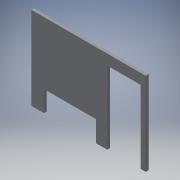
# Autodesk Inventor part: CANIMDWall
Saved by Autodesk Inventor 2017 (Build 210142000, 142)
## iProperties
Created: 2017-03-28
Part Number: CANIMDWall
Material: Generic
Document SubType Name: Modeling
Designer: hoeflinc
Density: 1 g/cm^3
Appearance: Default
Quantity: 1
Author: hoeflinc
Autodesk Inventor part; units mm, degrees
ref_plane "YZ Plane" through (0, 0, 0) normal (1, 0, 0) x (0, 1, 0)
ref_plane "XZ Plane" through (0, 0, 0) normal (0, 1, 0) x (-1, 0, 0)
ref_plane "XY Plane" through (0, 0, 0) normal (0, 0, 1) x (1, 0, 0)
sketch "Sketch1" plane through (0, 0, 0) normal (0, 0, 1) x (1, 0, 0)
  line L0 (0, 0) -> (139.7, 0)
  line L1 (139.7, 0) -> (139.7, 101.6)
  line L2 (139.7, 101.6) -> (0, 101.6)
  line L3 (0, 101.6) -> (0, 0)
  dimension "d0" = 139.7
  dimension "d1" = 101.6
  constraints: 8 end point, 2 parallel, 1 horizontal, 1 perpendicular
  measures "d0" distance of L1.end L2.end
  measures "d1" distance of L2.end L0.start
extrude "Extrusion1" add sketch "Sketch1" along normal blind 3.5
sketch "Sketch2" plane through (0, 0, 3.5) normal (0, 0, 1) x (1, 0, 0)
  line L0 (0, 0) -> (139.7, 0) projected
  line L1 (92.71, 0) -> (133.35, 0)
  line L2 (133.35, 0) -> (133.35, 88.9)
  line L3 (133.35, 88.9) -> (92.71, 88.9)
  line L4 (92.71, 88.9) -> (92.71, 0)
  line L5 (139.7, 0) -> (139.7, 101.6) projected
  dimension "d4" = 88.9
  dimension "d5" = 6.35
  dimension "d6" = 40.64
  constraints: 8 end point, 2 parallel, 1 horizontal, 1 perpendicular, 1 point on line
  measures "d4" distance of L3.end L1.start
  measures "d5" distance between parallel lines of L5 L2
  measures "d6" distance of L2.end L3.end
extrude "Extrusion2" cut sketch "Sketch2" against normal blind 3.5
sketch "Sketch3" plane through (0, 0, 3.5) normal (0, 0, 1) x (1, 0, 0)
  line L0 (15.24, 0) -> (78.74, 0)
  line L1 (78.74, 0) -> (78.74, 25.4)
  line L2 (78.74, 25.4) -> (15.24, 25.4)
  line L3 (15.24, 25.4) -> (15.24, 0)
  line L4 (133.35, 88.9) -> (133.35, 0) projected
  line L5 (133.35, 0) -> (139.7, 0) projected
  line L6 (139.7, 0) -> (139.7, 101.6) projected
  line L7 (139.7, 101.6) -> (0, 101.6) projected
  line L8 (0, 101.6) -> (0, 0) projected
  line L9 (0, 0) -> (92.71, 0) projected
  line L10 (92.71, 0) -> (92.71, 88.9) projected
  line L11 (92.71, 88.9) -> (133.35, 88.9) projected
  dimension "d9" = 25.4
  dimension "d10" = 13.97
  dimension "d11" = 63.5
  dimension "d12" = 0
  constraints: 8 end point, 2 parallel, 1 horizontal, 1 perpendicular
  measures "d9" distance of L0.end L1.end
  measures "d10" distance between parallel lines of L1 L10
  measures "d11" distance of L1.end L2.end
  measures "d12" distance between parallel lines of L9 L0
extrude "Extrusion3" cut sketch "Sketch3" against normal blind 3.5 contours L3 L2 L1 L0
body "Solid1"
